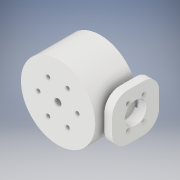
# Autodesk Inventor part: AA036
Saved by Autodesk Inventor 2017 SP1 (Build 210196100, 196)
## iProperties
Created: 2017-10-30
Part Number: AA036
Material: ABS Plastic
Document SubType Name: Modeling
Designer: Zach
Density: 1.06 g/cm^3
Appearance: CR White
Author: Zach
Autodesk Inventor part; units mm, degrees
ref_plane "YZ Plane" through (0, 0, 0) normal (1, 0, 0) x (0, 1, 0)
ref_plane "XZ Plane" through (0, 0, 0) normal (0, 1, 0) x (-1, 0, 0)
ref_plane "XY Plane" through (0, 0, 0) normal (0, 0, 1) x (1, 0, 0)
sketch "Sketch1" plane through (0, 0, 0) normal (0, 0, 1) x (1, 0, 0)
  circle A0 centre (0, 0) radius 47.5
  circle A1 centre (0, 0) radius 4.25
  circle A2 centre (25, 0) radius 2.5
  circle A3 centre (12.5, 21.6506) radius 2.5
  circle A4 centre (-12.5, 21.6506) radius 2.5
  circle A5 centre (-25, 0) radius 2.5
  circle A6 centre (-12.5, -21.6506) radius 2.5
  circle A7 centre (12.5, -21.6506) radius 2.5
  dimension "d0" = 95
  dimension "d1" = 8.5
  dimension "d2" = 5
  dimension "d3" = 25
  dimension "d6" = 360
  constraints: 8 centre point, 2 coincident, 1 horizontal alignment, 13 other
  measures "d0" diameter of A0
  measures "d1" diameter of A1
  measures "d2" diameter of A2
  measures "d3" distance of A2.centre point (0, 0)
extrude "Extrusion1" add sketch "Sketch1" along normal blind 54
ref_plane "Work Plane1" through (0, 0, 16) normal (0, 0, 1) x (1, 0, 0)
sketch "Sketch2" plane through (0, 0, 16) normal (0, 0, 1) x (1, 0, 0)
  circle A0 centre (0, 0) radius 47.5 projected
  line L0 (44.1588, 17.5) -> (51.1588, 17.5)
  line L1 (51.1588, 17.5) -> (51.1588, -17.5)
  line L2 (51.1588, -17.5) -> (44.1588, -17.5)
  line L3 (44.1588, -17.5) -> (44.1588, 17.5)
  point P0 (44.1588, 0)
  dimension "d11" = 7
  dimension "d12" = 35
  constraints: 8 end point, 2 parallel, 2 point on circle, 1 horizontal, 1 horizontal alignment, 1 midpoint, 1 perpendicular
  measures "d11" distance of L1.end L2.end
  measures "d12" distance of L0.end L1.end
extrude "Extrusion2" add sketch "Sketch2" along normal mid plane 25 contours A0 L0 L1 L2
sketch "Sketch3" plane through (51.1588, -17.5, 28.5) normal (1, 0, 0) x (0, 0, -1)
  line L0 (-17.5, 47.5) -> (42.5, 47.5)
  line L1 (42.5, 47.5) -> (42.5, -12.5)
  line L2 (42.5, -12.5) -> (-17.5, -12.5)
  line L3 (-17.5, -12.5) -> (-17.5, 47.5)
  line L4 (25, 35) -> (0, 35) projected
  line L5 (0, 0) -> (0, 35) projected
  line L6 (25, 0) -> (0, 0) projected
  line L7 (25, 35) -> (25, 0) projected
  line L8 (25, 35) -> (25, 0) projected
  point P0 (28.5, 17.5)
  point P1 (-17.5, 17.5)
  point P2 (25, 17.5)
  point P3 (12.5, 47.5)
  point P4 (12.5, 35)
  dimension "d15" = 60
  dimension "d16" = 60
  constraints: 8 end point, 4 midpoint, 2 parallel, 1 horizontal, 1 horizontal alignment, 1 perpendicular, 1 vertical alignment
  measures "d15" distance of L1.end L2.end
  measures "d16" distance of L0.end L1.end
extrude "Extrusion3" add sketch "Sketch3" along normal blind 10 contours L0 L1 L2 L3 | L7 L6 L5 L4
fillet "Fillet1" radius 20 4 edges at (56.1588, 30, 46) (56.1588, 30, -14) (56.1588, -30, -14) (56.1588, -30, 46)
sketch "Sketch4" plane through (61.1588, -17.5, 28.5) normal (1, 0, 0) x (0, 0, -1)
  line L0 (2.5, 32.5) -> (22.5, 32.5) construction
  line L1 (22.5, 32.5) -> (22.5, 2.5) construction
  line L2 (22.5, 2.5) -> (2.5, 2.5) construction
  line L3 (2.5, 2.5) -> (2.5, 32.5) construction
  line L4 (22.5, 47.5) -> (2.5, 47.5) projected
  line L5 (42.5, 7.5) -> (42.5, 27.5) projected
  circle A0 centre (2.5, 32.5) radius 2.5
  circle A1 centre (22.5, 32.5) radius 2.5
  circle A2 centre (2.5, 2.5) radius 2.5
  circle A3 centre (22.5, 2.5) radius 2.5
  point P0 (28.5, 17.5)
  point P1 (22.5, 17.5)
  point P2 (42.5, 17.5)
  point P3 (12.5, 32.5)
  point P4 (12.5, 47.5)
  dimension "d20" = 20
  dimension "d21" = 30
  dimension "d22" = 5
  dimension "d23" = 5
  dimension "d24" = 5
  dimension "d25" = 5
  constraints: 8 end point, 4 centre point, 4 coincident, 4 midpoint, 2 parallel, 1 horizontal, 1 horizontal alignment, 1 perpendicular, 1 vertical alignment
  measures "d20" distance of L1.end L2.end
  measures "d21" distance of L0.end L1.end
  measures "d22" diameter of A0
  measures "d23" diameter of A1
  measures "d24" diameter of A2
  measures "d25" diameter of A3
extrude "Extrusion4" cut sketch "Sketch4" against normal blind 30
sketch "Sketch5" plane through (61.1588, -17.5, 28.5) normal (1, 0, 0) x (0, 0, -1)
  circle A0 centre (12.5, 17.5) radius 14
  line L0 (42.5, 7.5) -> (42.5, 27.5) projected
  line L1 (2.5, -12.5) -> (22.5, -12.5) projected
  point P0 (28.5, 17.5)
  point P1 (12.5, -12.5)
  point P2 (42.5, 17.5)
  dimension "d28" = 28
  constraints: 2 midpoint, 1 centre point, 1 horizontal alignment, 1 vertical alignment
  measures "d28" diameter of A0
extrude "Extrusion5" cut sketch "Sketch5" against normal blind 13
equation "\"d26\" = d21"
body "Solid1"
